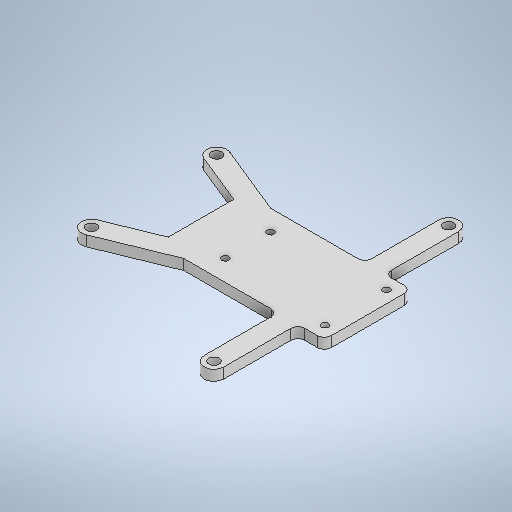
# Autodesk Inventor part: base_c
Saved by Autodesk Inventor 2025.2 (Build 292293000, 293)
## iProperties
Created: 2025-03-26
Part Number: base_c
Material: Generic
Document SubType Name: Modeling
Designer: cdavi
Density: 1 g/cm^3
Appearance: Default
Mass: 4.94389 g
Surface Area: 44.1455 cm^2
Volume: 4.94389 cm^3
Author: cdavi
Autodesk Inventor part; units mm, degrees
ref_plane "YZ Plane" through (0, 0, 0) normal (1, 0, 0) x (0, 1, 0)
ref_plane "XZ Plane" through (0, 0, 0) normal (0, 1, 0) x (-1, 0, 0)
ref_plane "XY Plane" through (0, 0, 0) normal (0, 0, 1) x (1, 0, 0)
sketch "Sketch1" plane through (0, 0, 0) normal (0, 1, 0) x (-1, 0, 0)
  line L0 (-29, 33.75) -> (29, 33.75)
  line L1 (29, 33.75) -> (29, -33.75)
  line L2 (29, -33.75) -> (-29, -33.75)
  line L3 (-29, -33.75) -> (-29, 33.75)
  line L4 (-29, 33.75) -> (29, -33.75) construction
  line L5 (29, 33.75) -> (-29, -33.75) construction
  line L6 (-32.5, 37.25) -> (32.5, 37.25)
  line L7 (32.5, -37.25) -> (-32.5, -37.25)
  line L8 (-32.5, -37.25) -> (-32.5, 37.25)
  line L9 (-32.5, 37.25) -> (32.5, -37.25) construction
  line L10 (32.5, 37.25) -> (-32.5, -37.25) construction
  line L11 (32.5, 37.25) -> (32.5, 5.9791)
  line L12 (32.5, -5.9791) -> (32.5, -37.25)
  line L13 (29, 0) -> (29, -18)
  circle A0 centre (29, -18) radius 1.5
  arc A1 (32.5, 5.9791) -> (32.5, -5.9791) centre (33, 0) ccw
  line L14 (32.5, -5.9791) -> (32.5, 5.9791)
  line L15 (33, 0) -> (-32.5, 0)
  line L16 (29, 0) -> (29, 18)
  circle A2 centre (29, 18) radius 1.5
  circle A3 centre (-22, -33.75) radius 1.5
  circle A4 centre (-22, 33.75) radius 1.5
  point P0 (0, 0)
  dimension "d1" = 58
  dimension "d3" = 3.5
  dimension "d31" = 67.5
  dimension "d32" = 3.5
  dimension "d33" = 18
  dimension "d34" = 3
  dimension "d57" = 51
  constraints: 34 end point, 6 midpoint, 5 centre point, 5 parallel, 3 perpendicular, 3 symmetric about line, 2 coincident, 2 horizontal, 2 point on circle, 2 point on line, 1 equal radius, 1 vertical, 3 other
  measures "d1" distance of L0.start L0.end
  measures "d3" distance between parallel lines of L7 L2
  measures "d31" distance of L0.end L1.end
  measures "d32" distance between parallel lines of L1 L11
  measures "d33" distance of L13.start L13.end
  measures "d34" diameter of A0
  measures "d57" distance from line of A3.centre L1
ref_plane "Work Plane1" through (0, 3, 0) normal (0, 1, 0) x (1, 0, 0)
extrude "Extrusion4" add sketch "Sketch1" along normal blind 3 contours A4 L0 L3 L15 L8 L6 L11 A1 L1 A2 | L0 L1 A2 A1 L15 L3 A4 | L15 A1 L1 A0 L2 A3 L3 | L3 L2 A3 L1 A0 A1 L12 L7 L8 L15
sketch "Sketch3" plane through (0, 3, 0) normal (0, 1, 0) x (1, 0, 0)
  circle A0 centre (-29, 18) radius 1.5 projected
  circle A1 centre (-29, 18) radius 2.85
  circle A2 centre (22, 33.75) radius 1.5
  line L0 (32.5, -37.25) -> (32.5, 37.25) projected
  line L1 (32.5, 0) -> (-15.5, 0)
  line L2 (-15.5, 0) -> (-15.5, 12.5)
  line L3 (-15.5, 12.5) -> (32.5, 12.5)
  line L4 (32.5, 12.5) -> (32.5, 0)
  line L5 (32.5, 0) -> (32.5, 12.5)
  line L6 (32.5, 0) -> (29, 0)
  line L7 (29, 0) -> (29, 8.825)
  line L8 (29, 8.825) -> (-2, 8.825)
  line L9 (-2, 8.825) -> (-2, 0)
  circle A3 centre (29, 8.825) radius 1
  line L10 (-15.5, 0) -> (-15.5, -12.5)
  line L11 (-15.5, -12.5) -> (32.5, -12.5)
  line L12 (32.5, -12.5) -> (32.5, 0)
  line L13 (29, 0) -> (29, -8.825)
  line L14 (29, -8.825) -> (-2, -8.825)
  line L15 (-2, -8.825) -> (-2, 0)
  circle A4 centre (29, -8.825) radius 1
  line L16 (32.5, 26) -> (32.5, 12.5)
  line L17 (-29, 18) -> (-15.5, 12.5)
  line L18 (-30.0753, 15.3606) -> (-15.5, 9.4226)
  line L19 (-27.9247, 20.6394) -> (-13.3494, 14.7013)
  line L20 (32.5, 26) -> (32.5, 12.5)
  line L21 (-13.3494, 14.7013) -> (-7.9463, 12.5)
  circle A5 centre (-29, -18) radius 2.85
  line L22 (-29, -18) -> (-15.5, -12.5)
  line L23 (-30.0753, -15.3606) -> (-15.5, -9.4226)
  line L24 (-27.9247, -20.6394) -> (-13.3494, -14.7013)
  line L25 (-13.3494, -14.7013) -> (-7.9463, -12.5)
  circle A6 centre (22, 33.75) radius 2.85
  line L26 (32.5, 12.5) -> (15.5, 12.5)
  circle A7 centre (-2, 6.5) radius 1
  circle A8 centre (-2, -6.5) radius 1
  circle A9 centre (22, 33.75) radius 1.5 projected
  circle A10 centre (22, -33.75) radius 1.5
  circle A11 centre (22, -33.75) radius 2.85
  circle A12 centre (22, -33.75) radius 1.5
  line L27 (24.85, 33.75) -> (24.85, 12.5)
  line L28 (19.15, 33.75) -> (19.15, 12.5)
  line L29 (24.85, -33.75) -> (24.85, -12.5)
  line L30 (19.15, -33.75) -> (19.15, -12.5)
  point P0 (0, 0)
  point P1 (-27.9247, 20.6394)
  point P2 (-27.9247, -20.6394)
  point P3 (-7.9463, -12.5)
  point P4 (32.5, -12.5)
  point P5 (19.15, -12.5)
  point P6 (19.15, 12.5)
  dimension "d37" = 5.7
  dimension "d38" = 48
  dimension "d39" = 12.5
  dimension "d40" = 3.5
  dimension "d41" = 8.825
  dimension "d42" = 31
  dimension "d44" = 2
  dimension "d48" = 5.7
  dimension "d49" = 17
  dimension "d56" = 6.5
  constraints: 60 end point, 22 symmetric about line, 10 point on line, 9 centre point, 6 coincident, 4 perpendicular, 3 collinear, 3 horizontal, 2 equal radius, 2 parallel, 2 point on circle, 2 tangent, 2 vertical, 1 concentric, 1 midpoint, 12 other
  measures "d38" distance of L1.start L1.end
  measures "d39" distance of L1.end L2.end
  measures "d40" distance of L1.start L6.end
  measures "d41" distance of L6.end L7.end
  measures "d42" distance of L7.end L8.end
  measures "d44" diameter of A3
  measures "d48" diameter of A6
  measures "d49" distance of L3.end L26.end
  measures "d56" distance from line of A7.centre L1
extrude "Extrusion6" cut sketch "Sketch3" against normal blind 48 contours A0 | A1 | A1 L19 L21 L3 L17 | L17 L2 L18 A1 | L3 L0 L1 L7 A3 L8 L9 A7 L2 | L1 L15 A8 L14 A4 L13 L0 L11 L10 | L9 A7 L8 A3 L7 L1 | L1 L13 A4 L14 L15 A8 | L10 L22 A5 L23 | L28 A6 L27 L3 | L11 L25 L24 A5 L22 | A5 | A6 | L11 L29 A11 L30 | A11 | A2 | A10 keep common part
fillet "Fillet3" radius 2 6 edges at (32.5, 1.5, 12.5) (32.5, 1.5, -12.5) (24.85, 1.5, 12.5) (19.15, 1.5, 12.5) (24.85, 1.5, -12.5) (19.15, 1.5, -12.5)
equation "\"d53\" = d38"
body "Solid2"
